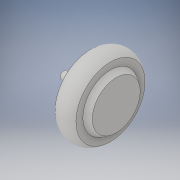
# Autodesk Inventor part: Wheel
Saved by Autodesk Inventor 2019.3 (Build 233278000, 278)
## iProperties
Created: 2019-01-27
Part Number: Wheel
Material: Generic
Document SubType Name: Modeling
Designer: mark
Density: 1 g/cm^3
Appearance: Default
Author: mark
Autodesk Inventor part; units mm, degrees
ref_plane "YZ Plane" through (0, 0, 0) normal (1, 0, 0) x (0, 1, 0)
ref_plane "XZ Plane" through (0, 0, 0) normal (0, 1, 0) x (-1, 0, 0)
ref_plane "XY Plane" through (0, 0, 0) normal (0, 0, 1) x (1, 0, 0)
sketch "Sketch4" plane through (0, 0, 0) normal (0, 0, 1) x (1, 0, 0)
  line L0 (0, 0) -> (0, 7.95)
  line L1 (0, 7.95) -> (51.5, 7.95)
  line L2 (51.5, 7.95) -> (51.5, 16.65)
  line L3 (51.5, 16.65) -> (56.5, 23.25)
  line L4 (56.5, 23.25) -> (56.5, 75)
  arc A0 (101.5, 75) -> (56.5, 75) centre (79, 54.6875) ccw
  line L5 (101.5, 75) -> (101.5, 60)
  line L6 (101.5, 60) -> (114, 52)
  line L7 (114, 52) -> (114, 0)
  line L8 (114, 0) -> (0, 0)
  line L9 (101.5, 75) -> (56.5, 75)
  point P0 (79, 75)
  dimension "d6" = 7.95
  dimension "d7" = 16.65
  dimension "d8" = 23.25
  dimension "d9" = 75
  dimension "d10" = 85
  dimension "d11" = 15
  dimension "d12" = 8
  dimension "d13" = 51.5
  dimension "d14" = 5
  dimension "d15" = 45
  dimension "d16" = 12.5
  constraints: 20 end point, 6 perpendicular, 2 horizontal, 2 point on circle, 1 centre point, 1 midpoint
  measures "d6" distance between parallel lines of L1 L8
  measures "d7" distance from line of L2.end L8
  measures "d8" distance from line of L3.end L8
  measures "d9" distance from line of L4.end L8
  measures "d11" distance of L5.end L5.start
  measures "d12" vertical distance of L6.end L5.end
  measures "d13" distance between parallel lines of L2 L0
  measures "d14" distance between parallel lines of L4 L2
  measures "d15" distance between parallel lines of L5 L4
  measures "d16" distance between parallel lines of L5 L7
revolve "Revolution1" add sketch "Sketch4" angle 360 about axis through (114, 0, 0) along (-1, 0, 0)
sketch "Sketch5" plane through (0, 0, 0) normal (-1, 0, 0) x (0, 0, 1)
  line L0 (-5.3, -5.9256) -> (-5.3, 5.9256)
  circle A0 centre (0, 0) radius 7.95 projected
  circle A1 centre (0, 0) radius 7.95 projected
  arc A2 (-5.3, 5.9256) -> (-5.3, -5.9256) centre (0, 0) ccw
  point P0 (0, 0)
  point P1 (-7.95, 0)
  dimension "d18" = 5.3
  constraints: 7 point on circle, 2 end point, 1 centre point, 1 vertical
  measures "d18" distance from line of L0 point (0, 0)
extrude "Extrusion3" cut sketch "Sketch5" against normal blind 46.5 contours A0 L0 picked at (-6.5836, -0.1596)
sketch "Sketch6" plane through (0, 0, 0) normal (-1, 0, 0) x (0, 0, 1)
  circle A0 centre (0, 0) radius 7.95 projected
  line L0 (-5.3, -5.9256) -> (-5.3, 5.9256)
  arc A1 (-5.3, 5.9256) -> (-5.3, -5.9256) centre (0, 0) ccw
  point P0 (0, 0)
  point P1 (-7.95, 0)
  constraints: 4 point on circle, 2 end point, 1 centre point
extrude "Extrusion4" add sketch "Sketch6" against normal blind 2.5
sketch "Sketch7" plane through (0, 0, 0) normal (-1, 0, 0) x (0, 0, 1)
  circle A0 centre (0, 0) radius 3.75
  point P0 (0, 0)
  dimension "d23" = 7.5
  constraints: 1 centre point, 1 coincident
  measures "d23" diameter of A0
extrude "Extrusion5" cut sketch "Sketch7" against normal up to surface (56.5 mm away)
body "Solid2"
